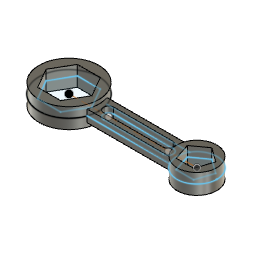
spanner(ex 2) (Autodesk Fusion 360 design; units mm, degrees)
Autodesk Fusion 360 part; units mm, degrees
sketch "Sketch1" plane through (0, 0, 0) normal (0, 0, 1) x (1, 0, 0)
  circle A0 centre (0, 0) radius 30
  circle A1 centre (129, 0) radius 20
  line L0 (0, 0) -> (0, 0)
  line L1 (0, 0) -> (0, 0)
  line L2 (0, 0) -> (0, 0)
  line L3 (0, 0) -> (0, 0)
  line L4 (0, 0) -> (0, 0)
  line L5 (0, 0) -> (0, 0)
  line L6 (-11.547, 20) -> (-23.094, 0)
  line L7 (-23.094, 0) -> (-11.547, -20)
  line L8 (-11.547, -20) -> (11.547, -20)
  line L9 (11.547, -20) -> (23.094, 0)
  line L10 (23.094, 0) -> (11.547, 20)
  line L11 (11.547, 20) -> (-11.547, 20)
  line L12 (129, 15) -> (114.7342, 4.6353)
  line L13 (114.7342, 4.6353) -> (120.1832, -12.1353)
  line L14 (120.1832, -12.1353) -> (137.8168, -12.1353)
  line L15 (137.8168, -12.1353) -> (143.2658, 4.6353)
  line L16 (143.2658, 4.6353) -> (129, 15)
  line L17 (0, 0) -> (129, 0) construction
  line L18 (28.2843, 10) -> (111.6795, 10)
  line L19 (28.2843, -10) -> (111.6795, -10)
  line L20 (40, 5) -> (100, 5)
  line L21 (40, -5) -> (100, -5)
  arc A2 (40, 5) -> (40, -5) centre (40, 0) ccw
  arc A3 (100, -5) -> (100, 5) centre (100, 0) ccw
  point P0 (129, 0)
  dimension "d1" = 60
  dimension "d2" = 129
  dimension "d3" = 40
  dimension "d4" = 20
  dimension "d5" = 15
  constraint coincident A0.centre L0.start
  constraint coincident P0 A1.centre
  constraint horizontal L18
  constraint horizontal L19
  constraint coincident A0 L18.start
  constraint coincident A0 L19.start
  constraint coincident A1 L19.end
  constraint coincident A1 L18.end
  constraint tangent L20 A2
  constraint tangent L20 A3
  measures "d1" diameter of A0
  measures "d2" distance of A0.centre P0
  measures "d3" diameter of A1
  measures "d4" distance of A0.centre L11
  measures "d5" distance of L12.start P0
extrude "Extrude1" add sketch "Sketch1" along normal mid plane 20 contours A0 | A1 makes body 1 at (25.0013, -16.5811, 3.3333) makes body 2 at (148.9006, -1.9914, -3.3333)
extrude "Extrude2" add sketch "Sketch1" along normal mid plane 12 contours A0 A1 L18 L19 bodies 1 2
sketch "Sketch3" plane through (0, 0, 0) normal (0, 0, 1) x (1, 0, 0)
sketch "Sketch4" plane through (0, 0, 0) normal (0, 0, 1) x (1, 0, 0)
